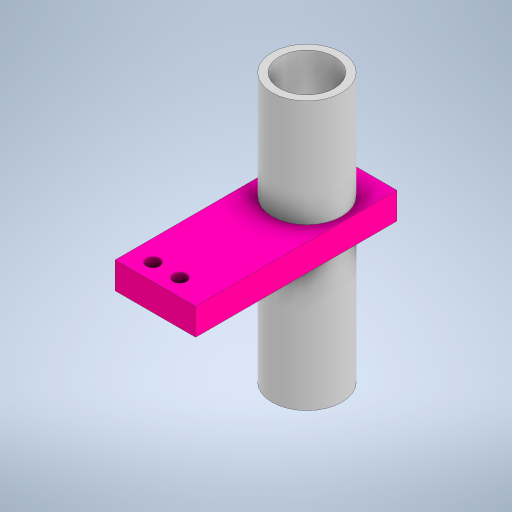
# Autodesk Inventor part: Flip up and down motion motor mount
Saved by Autodesk Inventor 2023.1 (Build 271208000, 208)
## iProperties
Created: 2022-12-20
Part Number: Flip up and down motion motor mount
Material: Generic
Document SubType Name: Modeling
Designer: shubh
Density: 1 g/cm^3
Appearance: Default
Author: shubh
Autodesk Inventor part; units mm, degrees
ref_plane "YZ Plane" through (0, 0, 0) normal (1, 0, 0) x (0, 1, 0)
ref_plane "XZ Plane" through (0, 0, 0) normal (0, 1, 0) x (-1, 0, 0)
ref_plane "XY Plane" through (0, 0, 0) normal (0, 0, 1) x (1, 0, 0)
sketch "Sketch1" plane through (0, 0, 0) normal (0, 1, 0) x (-1, 0, 0)
  line L0 (0, 0) -> (-38.1, 0)
  line L1 (-38.1, 0) -> (-38.1, -82.55)
  line L2 (-38.1, -82.55) -> (0, -82.55)
  line L3 (0, -82.55) -> (0, 0)
  circle A0 centre (-22.6822, 4.7752) radius 3.175
  circle A1 centre (-9.9822, 4.7752) radius 3.175
  line L4 (0, 0) -> (-38.1, 0)
  line L5 (-38.1, 0) -> (-38.1, 12.7)
  line L6 (-38.1, 12.7) -> (0, 12.7)
  line L7 (0, 12.7) -> (0, 0)
  dimension "d0" = 38.1
  dimension "d1" = 82.55
  dimension "d24" = 6.35
  dimension "d25" = 15.4178
  dimension "d27" = 6.35
  dimension "d28" = 12.7
  dimension "d29" = 12.7
  dimension "d30" = 7.9248
  constraints: 16 end point, 4 parallel, 2 centre point, 2 horizontal, 2 perpendicular
  measures "d0" distance of L1.end L2.end
  measures "d1" distance of L0.end L1.end
  measures "d24" diameter of A0
  measures "d25" distance from line of A0.centre L1
  measures "d27" diameter of A1
  measures "d28" distance of A1.centre A0.centre
  measures "d29" distance of L4.end L5.end
  measures "d30" distance from line of L6 A0.centre
extrude "Extrusion1" add sketch "Sketch1" along normal blind 12.7
sketch "Sketch2" plane through (0, 12.7, 0) normal (0, 1, 0) x (1, 0, 0)
  circle A0 centre (19.3548, 58.7375) radius 16.51
  line L0 (0, 82.55) -> (0, 0) projected
  line L1 (38.1, 82.55) -> (0, 82.55) projected
  point P0 (9.6774, 7.9375)
  dimension "d8" = 33.02
  dimension "d23" = 9.6774
  constraints: 1 centre point
  measures "d8" diameter of A0
  measures "d23" horizontal distance of A0.centre point (9.677, 7.938)
extrude "Extrusion2" add sketch "Sketch2" along normal blind 50.8 and the other way blind 76.2
sketch "Sketch3" plane through (19.3548, 63.5, -58.7375) normal (0, 1, 0) x (1, 0, 0)
  circle A0 centre (0, 0) radius 13.0175
  point P0 (-19.3548, -58.7375)
  dimension "d17" = 26.035
  constraints: 1 centre point
  measures "d17" diameter of A0
extrude "Extrusion3" cut sketch "Sketch3" against normal blind 41.91
sketch "Sketch4" plane through (19.3548, 21.59, -58.7375) normal (0, 1, 0) x (1, 0, 0)
  circle A0 centre (0, 0) radius 16
  point P0 (-19.3548, -58.7375)
  dimension "d20" = 31.9999
  constraints: 1 centre point
  measures "d20" diameter of A0
extrude "Extrusion4" cut sketch "Sketch4" against normal blind 59.69
body "Solid1"
